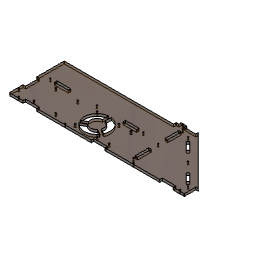
Side Plate Left (Autodesk Fusion 360 design; units mm, degrees)
Autodesk Fusion 360 part; units mm, degrees
note: some values were not read from the file. Set by a fixed rule: which sketch regions a step uses.
sketch "Sketch1" plane through (0, 0, 0) normal (0, 0, 1) x (1, 0, 0)
  line L0 (0, 0) -> (320, 0)
  line L1 (320, 0) -> (320, 10)
  line L2 (320, 10) -> (225, 105)
  line L3 (225, 105) -> (200, 105)
  line L4 (200, 105) -> (200, 100.25)
  line L5 (200, 100.25) -> (0, 100.25)
  line L6 (0, 100.25) -> (0, 0)
  line L7 (-10, 62.25) -> (295, 62.25) construction
  line L8 (-10, 57.75) -> (295, 57.75) construction
  line L9 (-10, 4.5) -> (325, 4.5) construction
  line L10 (9.1552, 60) -> (314.1552, 60) construction
  line L11 (325.1257, 2.25) -> (-10, 2.25) construction
  line L12 (25, 105) -> (25, -5) construction
  line L13 (50, 105) -> (50, -5) construction
  line L14 (175, 105) -> (175, -5) construction
  line L15 (150, 105) -> (150, -5) construction
  line L16 (4.5, 110) -> (4.5, -5) construction
  line L17 (150, 62.25) -> (175, 62.25)
  line L18 (175, 62.25) -> (175, 57.75)
  line L19 (175, 57.75) -> (150, 57.75)
  line L20 (150, 57.75) -> (150, 62.25)
  line L21 (25, 62.25) -> (50, 62.25)
  line L22 (50, 62.25) -> (50, 57.75)
  line L23 (50, 57.75) -> (25, 57.75)
  line L24 (25, 57.75) -> (25, 62.25)
  line L25 (25, 4.5) -> (50, 4.5)
  line L26 (50, 4.5) -> (50, 0)
  line L27 (50, 0) -> (25, 0)
  line L28 (25, 0) -> (25, 4.5)
  line L29 (150, 4.5) -> (175, 4.5)
  line L30 (175, 4.5) -> (175, 0)
  line L31 (175, 0) -> (150, 0)
  line L32 (150, 0) -> (150, 4.5)
  line L33 (300, -5) -> (300, 105) construction
  line L34 (275, 105) -> (275, -5) construction
  line L35 (275, 4.5) -> (300, 4.5)
  line L36 (300, 4.5) -> (300, 0)
  line L37 (300, 0) -> (275, 0)
  line L38 (275, 0) -> (275, 4.5)
  line L39 (0, 25) -> (4.5, 25)
  line L40 (4.5, 25) -> (4.5, 50)
  line L41 (4.5, 50) -> (0, 50)
  line L42 (0, 50) -> (0, 25)
  line L43 (215, 110) -> (215, -5) construction
  line L44 (219.5, 110) -> (219.5, -5) construction
  line L45 (250, 95) -> (182.1863, 95) construction
  line L46 (250, 70) -> (182.1863, 70) construction
  line L47 (250, 15) -> (182.1863, 15) construction
  line L48 (250, 40) -> (182.1863, 40) construction
  line L49 (219.5, 15) -> (215, 15)
  line L50 (215, 15) -> (215, 40)
  line L51 (215, 40) -> (219.5, 40)
  line L52 (219.5, 40) -> (219.5, 15)
  line L53 (219.5, 70) -> (215, 70)
  line L54 (215, 70) -> (215, 95)
  line L55 (215, 95) -> (219.5, 95)
  line L56 (219.5, 95) -> (219.5, 70)
  line L57 (217.25, 110) -> (217.25, -5) construction
  circle A0 centre (217.25, 100) radius 1.15
  circle A1 centre (217.25, 55) radius 1.15
  circle A2 centre (217.25, 10) radius 1.15
  circle A3 centre (185, 60) radius 1.15
  circle A4 centre (100, 60) radius 1.15
  circle A5 centre (15, 60) radius 1.15
  circle A6 centre (15, 2.25) radius 1.15
  circle A7 centre (100, 2.25) radius 1.15
  circle A8 centre (225, 2.25) radius 1.15
  circle A9 centre (310, 2.25) radius 1.15
  line L58 (329.3164, -5.6804) -> (209.3319, 114.3041) construction
  line L59 (242.2183, 87.7817) -> (239.0363, 84.5998)
  line L60 (256.3604, 73.6396) -> (253.1784, 70.4576)
  line L61 (291.7157, 38.2843) -> (288.5337, 35.1023)
  line L62 (305.8579, 24.1421) -> (302.6759, 20.9602)
  line L63 (239.0363, 84.5998) -> (253.1784, 70.4576)
  line L64 (288.5337, 35.1023) -> (302.6759, 20.9602)
  line L65 (330.1331, -3.3151) -> (213.3936, 113.4244) construction
  circle A10 centre (311.3379, 15.4801) radius 1.15
  circle A11 centre (272.4471, 54.371) radius 1.15
  circle A12 centre (233.5562, 93.2618) radius 1.15
  line L66 (2.25, -5) -> (2.25, 105) construction
  circle A13 centre (2.25, 15) radius 1.15
  line L67 (204.9, 105) -> (214.9, 105)
  line L68 (214.9, 105) -> (214.9, 109.5)
  line L69 (214.9, 109.5) -> (204.9, 109.5)
  line L70 (204.9, 109.5) -> (204.9, 105)
  line L71 (204.9, 107.25) -> (215.1, 107.25) construction
  circle A14 centre (210, 107.25) radius 1.15
  line L72 (236, 105) -> (225, 105)
  line L73 (236, 105) -> (236, 109.5)
  line L74 (320, 0) -> (331, 0)
  line L75 (331, 0) -> (331, 10)
  line L76 (331, 10) -> (331, 14.5)
  line L77 (331, 14.5) -> (236, 109.5)
  line L78 (320, 10) -> (320, 25.5)
  line L79 (340, 30) -> (285, 30)
  line L80 (75, 10) -> (35, 10) construction
  line L81 (35, 10) -> (35, 50) construction
  line L82 (35, 50) -> (75, 50) construction
  line L83 (75, 50) -> (75, 10) construction
  line L84 (75, 10) -> (35, 50) construction
  line L85 (35, 10) -> (75, 50) construction
  circle A15 centre (75, 50) radius 1.45
  circle A16 centre (75, 10) radius 1.45
  circle A17 centre (35, 50) radius 1.45
  circle A18 centre (35, 10) radius 1.45
  line L86 (320, 21) -> (324.5, 21)
  line L87 (155, 5.5) -> (105, 5.5) construction
  line L88 (105, 5.5) -> (105, 55.5) construction
  line L89 (105, 55.5) -> (155, 55.5) construction
  line L90 (155, 55.5) -> (155, 5.5) construction
  line L91 (155, 5.5) -> (105, 55.5) construction
  line L92 (105, 5.5) -> (155, 55.5) construction
  line L93 (150, 10.5) -> (110, 10.5) construction
  line L94 (110, 10.5) -> (110, 50.5) construction
  line L95 (110, 50.5) -> (150, 50.5) construction
  line L96 (150, 50.5) -> (150, 10.5) construction
  line L97 (150, 10.5) -> (110, 50.5) construction
  line L98 (110, 10.5) -> (150, 50.5) construction
  circle A19 centre (150, 50.5) radius 1.6
  circle A20 centre (110, 50.5) radius 1.6
  circle A21 centre (150, 10.5) radius 1.6
  circle A22 centre (110, 10.5) radius 1.6
  circle A23 centre (130, 30.5) radius 12.5
  circle A24 centre (130, 30.5) radius 23.5
  line L99 (132.5, 35.5) -> (127.5, 35.5)
  line L100 (127.5, 35.5) -> (127.5, 55.5)
  line L101 (127.5, 55.5) -> (132.5, 55.5)
  line L102 (132.5, 55.5) -> (132.5, 35.5)
  line L103 (132.5, 35.5) -> (127.5, 55.5) construction
  line L104 (127.5, 35.5) -> (132.5, 55.5) construction
  line L105 (107.0994, 20.1651) -> (124.4199, 30.1651)
  line L106 (109.5994, 15.8349) -> (107.0994, 20.1651)
  line L107 (126.9199, 25.8349) -> (109.5994, 15.8349)
  line L108 (124.4199, 30.1651) -> (126.9199, 25.8349)
  line L109 (124.4199, 30.1651) -> (109.5994, 15.8349) construction
  line L110 (126.9199, 25.8349) -> (107.0994, 20.1651) construction
  line L111 (150.4006, 15.8349) -> (133.0801, 25.8349)
  line L112 (152.9006, 20.1651) -> (150.4006, 15.8349)
  line L113 (135.5801, 30.1651) -> (152.9006, 20.1651)
  line L114 (133.0801, 25.8349) -> (135.5801, 30.1651)
  line L115 (133.0801, 25.8349) -> (152.9006, 20.1651) construction
  line L116 (135.5801, 30.1651) -> (150.4006, 15.8349) construction
  line L117 (183.5, 7) -> (160.5, 7) construction
  line L118 (160.5, 7) -> (160.5, 54) construction
  line L119 (160.5, 54) -> (183.5, 54) construction
  line L120 (183.5, 54) -> (183.5, 7) construction
  line L121 (183.5, 7) -> (160.5, 54) construction
  line L122 (160.5, 7) -> (183.5, 54) construction
  line L123 (172, 62) -> (172, 11) construction
  circle A25 centre (172, 50.5) radius 1.6
  circle A26 centre (172, 10.5) radius 1.6
  point P0 (55, 30)
  point P1 (130, 30.5)
  point P2 (130, 30.5)
  point P3 (130, 45.5)
  point P4 (172, 30.5)
  dimension "d2" = 38
  dimension "d3" = 4.5
  dimension "d4" = 4.5
  dimension "d5" = 2.25
  dimension "d6" = 2.25
  dimension "d7" = 4.5
  dimension "d8" = 25
  dimension "d11" = 200
  dimension "d12" = 15
  dimension "d13" = 4.5
  dimension "d15" = 2.25
  dimension "d16" = 2.3
  dimension "d17" = 2.3
  dimension "d18" = 2.3
  dimension "d19" = 15
  dimension "d20" = 5
  dimension "d21" = 5
  dimension "d22" = 2.3
  dimension "d23" = 10
  dimension "d24" = 2.3
  dimension "d25" = 2.3
  dimension "d26" = 10
  dimension "d27" = 50
  dimension "d28" = 2.3
  dimension "d29" = 2.3
  dimension "d30" = 2.3
  dimension "d31" = 50
  dimension "d32" = 50
  dimension "d33" = 10
  dimension "d34" = 2.3
  dimension "d35" = 10
  dimension "d36" = 4.5
  dimension "d37" = 20
  dimension "d38" = 20
  dimension "d41" = 10
  dimension "d42" = 20
  dimension "d43" = 120
  dimension "d44" = 50
  dimension "d45" = 2.25
  dimension "d46" = 2.3
  dimension "d47" = 2.3
  dimension "d48" = 2.3
  dimension "d49" = 10
  dimension "d50" = 10
  dimension "d51" = 25
  dimension "d52" = 2.25
  dimension "d53" = 2.3
  dimension "d65" = 25
  dimension "d66" = 15
  dimension "d68" = 60
  dimension "d78" = 10
  dimension "d79" = 4.5
  dimension "d80" = 2.3
  dimension "d83" = 10
  dimension "d84" = 4.5
  dimension "d85" = 10
  dimension "d86" = 4.5
  dimension "d89" = 30
  dimension "d92" = 40
  dimension "d93" = 40
  dimension "d94" = 30
  dimension "d95" = 55
  dimension "d96" = 2.9
  dimension "d97" = 2.9
  dimension "d98" = 2.9
  dimension "d99" = 2.9
  dimension "d100" = 11
  dimension "d101" = 135
  dimension "d104" = 4.5
  dimension "d105" = 50
  dimension "d106" = 50
  dimension "d107" = 26
  dimension "d108" = 30
  dimension "d109" = 40
  dimension "d110" = 40
  dimension "d111" = 3.2
  dimension "d112" = 3.2
  dimension "d113" = 3.2
  dimension "d114" = 3.2
  dimension "d115" = 25
  dimension "d116" = 47
  dimension "d117" = 5
  dimension "d118" = 20
  dimension "d120" = 360
  dimension "d121" = 23
  dimension "d122" = 47
  dimension "d123" = 42
  dimension "d124" = 3.2
  dimension "d125" = 3.2
  dimension "d126" = 20
  dimension "d127" = 20
  constraint coincident L0.start L6.end
  constraint horizontal L0
  constraint perpendicular L0 L1
  constraint parallel L0 L3
  constraint perpendicular L3 L4
  constraint perpendicular L4 L5
  constraint perpendicular L0 L6
  constraint horizontal L7
  constraint horizontal L8
  constraint parallel L0 L9
  constraint parallel L8 L10
  constraint parallel L9 L11
  constraint perpendicular L5 L12
  constraint perpendicular L5 L13
  constraint perpendicular L11 L14
  constraint perpendicular L5 L15
  constraint perpendicular L9 L16
  constraint horizontal L17
  constraint vertical L18
  constraint horizontal L19
  constraint vertical L20
  constraint coincident L14 L18.end
  constraint coincident L8 L18.end
  constraint coincident L15 L17.start
  constraint coincident L7 L17.start
  constraint horizontal L21
  constraint vertical L22
  constraint horizontal L23
  constraint vertical L24
  constraint coincident L8 L22.end
  constraint coincident L13 L22.end
  constraint coincident L12 L21.start
  constraint coincident L7 L21.start
  constraint horizontal L25
  constraint vertical L26
  constraint horizontal L27
  constraint vertical L28
  constraint coincident L13 L26.end
  constraint coincident L0 L26.end
  constraint coincident L12 L25.start
  constraint coincident L9 L25.start
  constraint horizontal L29
  constraint vertical L30
  constraint horizontal L31
  constraint vertical L32
  constraint coincident L0 L30.end
  constraint coincident L14 L30.end
  constraint coincident L15 L29.start
  constraint coincident L9 L29.start
  constraint perpendicular L11 L33
  constraint perpendicular L0 L34
  constraint horizontal L35
  constraint vertical L36
  constraint horizontal L37
  constraint vertical L38
  constraint coincident L33 L36.end
  constraint coincident L0 L36.end
  constraint coincident L34 L35.start
  constraint coincident L9 L35.start
  constraint horizontal L39
  constraint vertical L40
  constraint horizontal L41
  constraint vertical L42
  constraint coincident L6 L39.start
  constraint perpendicular L0 L43
  constraint perpendicular L0 L44
  constraint perpendicular L43 L45
  constraint perpendicular L43 L46
  constraint perpendicular L43 L47
  constraint perpendicular L44 L48
  constraint horizontal L49
  constraint vertical L50
  constraint horizontal L51
  constraint vertical L52
  constraint coincident L43 L50.end
  constraint coincident L48 L50.end
  constraint coincident L44 L49.start
  constraint coincident L47 L49.start
  constraint horizontal L53
  constraint vertical L54
  constraint horizontal L55
  constraint vertical L56
  constraint coincident L45 L54.end
  constraint coincident L43 L54.end
  constraint coincident L46 L53.start
  constraint coincident L44 L53.start
  constraint parallel L43 L57
  constraint coincident L57 A0.centre
  constraint coincident L57 A1.centre
  constraint coincident L57 A2.centre
  constraint coincident L10 A3.centre
  constraint coincident L10 A4.centre
  constraint coincident L10 A5.centre
  constraint coincident L11 A6.centre
  constraint coincident L11 A7.centre
  constraint coincident L11 A8.centre
  constraint coincident L11 A9.centre
  constraint parallel L2 L58
  constraint coincident L2 L59.start
  constraint coincident L58 L59.end
  constraint perpendicular L58 L59
  constraint coincident L2 L60.start
  constraint coincident L58 L60.end
  constraint perpendicular L58 L60
  constraint coincident L2 L61.start
  constraint coincident L58 L61.end
  constraint perpendicular L58 L61
  constraint coincident L2 L62.start
  constraint coincident L58 L62.end
  constraint perpendicular L58 L62
  constraint parallel L58 L65
  constraint coincident L65 A10.centre
  constraint coincident L65 A11.centre
  constraint coincident L65 A12.centre
  constraint perpendicular L0 L66
  constraint coincident L66 A13.centre
  constraint horizontal L67
  constraint vertical L68
  constraint horizontal L69
  constraint vertical L70
  constraint coincident L3 L67.start
  constraint midpoint L70 L71.start
  constraint perpendicular L70 L71
  constraint midpoint L71 A14.centre
  constraint perpendicular L72 L73
  constraint perpendicular L1 L74
  constraint perpendicular L74 L75
  constraint parallel L75 L76
  constraint coincident L77 L78.end
  constraint parallel L1 L78
  constraint perpendicular L33 L79
  constraint horizontal L80
  constraint perpendicular L80 L81
  constraint parallel L80 L82
  constraint parallel L81 L83
  constraint coincident L84 P0
  constraint coincident L85 P0
  constraint coincident L82.end L83.start
  constraint coincident L80.start L83.end
  constraint coincident L81.end L82.start
  constraint coincident L80.end L81.start
  constraint collinear L3 L72
  constraint coincident L78 L86.start
  constraint perpendicular L78 L86
  constraint horizontal L87
  constraint perpendicular L87 L88
  constraint parallel L87 L89
  constraint parallel L88 L90
  constraint coincident L91 P2
  constraint coincident L92 P2
  constraint horizontal L93
  constraint perpendicular L93 L94
  constraint parallel L93 L95
  constraint parallel L94 L96
  constraint coincident L97 P2
  constraint coincident L98 P2
  constraint coincident P2 P1
  constraint coincident L95.end L96.start
  constraint coincident L94.end L95.start
  constraint coincident L93.start L96.end
  constraint coincident L93.end L94.start
  constraint concentric A23 A24
  constraint horizontal L99
  constraint perpendicular L99 L100
  constraint parallel L99 L101
  constraint parallel L100 L102
  constraint coincident L103 P3
  constraint coincident L104 P3
  constraint collinear L89 L101
  constraint horizontal L117
  constraint perpendicular L117 L118
  constraint parallel L117 L119
  constraint parallel L118 L120
  constraint coincident L121 P4
  constraint coincident L122 P4
  constraint perpendicular L117 L123
  constraint coincident P4 L123
  constraint coincident L123 A25.centre
  constraint coincident L123 A26.centre
  measures "d2" distance of L5 L7
  measures "d3" distance of L7 L8
  measures "d4" distance of L0 L9
  measures "d5" distance of L7 L10
  measures "d6" distance of L9 L11
  measures "d7" distance of L6 L16
  measures "d8" distance of L39.start L41.end
  measures "d11" distance of L4.end L5.end
  measures "d12" distance of L4 L43
  measures "d13" distance of L43 L44
  measures "d15" distance of L43 L57
  measures "d16" diameter of A0
  measures "d17" diameter of A1
  measures "d18" diameter of A2
  measures "d19" distance of L48 A1.centre
  measures "d20" distance of L45 A0.centre
  measures "d21" distance of L47 A2.centre
  measures "d22" diameter of A3
  measures "d23" distance of L14 A3.centre
  measures "d24" diameter of A4
  measures "d25" diameter of A5 L31.end
  measures "d26" distance of L12 A5.centre
  measures "d27" distance of L13 A4.centre
  measures "d28" diameter of A6
  measures "d29" diameter of A7
  measures "d30" diameter of A8
  measures "d31" distance of L14 A8.centre
  measures "d32" distance of L13 A7.centre
  measures "d33" distance of L12 A6.centre
  measures "d34" diameter of A9
  measures "d35" distance of L33 A9.centre
  measures "d36" distance of L2 L58
  measures "d37" distance of L59 L60
  measures "d38" distance of L61 L62
  measures "d41" distance of L0.end L1.end
  measures "d42" distance of L1.end L62.start
  measures "d43" distance of L1 L4
  measures "d44" distance of L60.start L61.start
  measures "d45" distance of L2 L65
  measures "d46" diameter of A10
  measures "d47" diameter of A11
  measures "d48" diameter of A12
  measures "d49" distance of L62 A10.centre
  measures "d50" distance of L59 A12.centre
  measures "d51" distance of L61 A11.centre
  measures "d52" distance of L6 L66
  measures "d53" diameter of A13
  measures "d65" distance of L0 L39
  measures "d66" distance of L0 A13.centre
  measures "d68" distance of L0 L10
  measures "d78" distance of L67.start L67.end
  measures "d79" distance of L67.start L69.end
  measures "d80" diameter of A14
  measures "d83" distance of L4 A14.centre
  measures "d84" distance of L72.start L73.end
  measures "d85" distance of L74.end L75.end
  measures "d86" distance of L75.end L76.end
  measures "d89" distance of L74 L79
  measures "d92" distance of L81.end L82.end
  measures "d93" distance of L80.end L81.end
  measures "d94" distance of L0 P0
  measures "d95" distance of L6 P0
  measures "d96" diameter of A15
  measures "d97" diameter of A16
  measures "d98" diameter of A17
  measures "d99" diameter of A18
  measures "d100" distance of L2.end L72.start
  measures "d101" angle of L76 L77
  measures "d104" distance of L78.end L86.start
  measures "d105" distance of L88.end L89.end
  measures "d106" distance of L87.end L88.end
  measures "d107" distance of L9 P2
  measures "d108" distance of L83 L88
  measures "d109" distance of L94.end L95.end
  measures "d110" distance of L93.end L94.end
  measures "d111" diameter of A19
  measures "d112" diameter of A20
  measures "d113" diameter of A21
  measures "d114" diameter of A22
  measures "d115" diameter of A23
  measures "d116" diameter of A24
  measures "d117" distance of L100.end L101.end
  measures "d118" distance of L99.end L100.end
  measures "d121" distance of L118.end L119.end
  measures "d122" distance of L117.end L118.end
  measures "d123" distance of P2 P4
  measures "d124" diameter of A25
  measures "d125" diameter of A26
  measures "d126" distance of P4 A25.centre
  measures "d127" distance of P4 A26.centre
extrude "Extrude1" add sketch "Sketch1" along normal blind 4.5 contours L0 L1 L2 L3 L4 L5 L6 L25 L26 L28 L29 L30 L32 L35 L36 L38 L39 L40 L41 L59 L60 L61 L62 L63 L64 L67 | L3 L67 L68 L69 L70 | L2 L77 L78 L79 | L2 L72 L73 L77 L79 | L77 L78 L86 | A23 L99 L100 L102 L105 L107 L108 L111 L113 L114 | A23 L99 L100 L102 | A23 A24 L100 L102 | A23 A24 L111 L113 | A23 L111 L113 L114 | A24 L100 L101 L102 | A24 L111 L112 L113 | A23 L105 L107 L108 | A23 A24 L105 L107 | A24 L105 L106 L107
fillet "Fillet1" radius 0.5 6 edges at (320, 0, 2.25) (320, 10, 2.25) (225, 105, 2.25) (200, 105, 2.25) (0, 100.25, 2.25) (0, 0, 2.25)
sketch "Sketch2" plane through (0, 0, 4.5) normal (0, 0, 1) x (-1, 0, 0)
  arc A0 (0, -0.5) -> (-0.5, 0) centre (-0.5, -0.5) ccw
  line L0 (-0.5, 0) -> (-25, 0)
  line L1 (-25, 0) -> (-25, -4.5)
  line L2 (-25, -4.5) -> (-50, -4.5)
  line L3 (-50, -4.5) -> (-50, 0)
  line L4 (-50, 0) -> (-150, 0)
  line L5 (-150, 0) -> (-150, -4.5)
  line L6 (-150, -4.5) -> (-175, -4.5)
  line L7 (-175, -4.5) -> (-175, 0)
  line L8 (-175, 0) -> (-275, 0)
  line L9 (-275, 0) -> (-275, -4.5)
  line L10 (-275, -4.5) -> (-300, -4.5)
  line L11 (-300, -4.5) -> (-300, 0)
  line L12 (-300, 0) -> (-319.5, 0)
  line L13 (-305.8579, -24.1421) -> (-302.6759, -20.9602)
  line L14 (-302.6759, -20.9602) -> (-288.5338, -35.1023)
  line L15 (-288.5338, -35.1023) -> (-291.7157, -38.2843)
  line L16 (-291.7157, -38.2843) -> (-305.8579, -24.1421)
  line L17 (-256.3604, -73.6396) -> (-253.1784, -70.4576)
  line L18 (-253.1784, -70.4576) -> (-239.0363, -84.5998)
  line L19 (-239.0363, -84.5998) -> (-242.2183, -87.7818)
  line L20 (-242.2183, -87.7818) -> (-256.3604, -73.6396)
  arc A1 (-200.5, -105) -> (-200, -104.5) centre (-200.5, -104.5) ccw
  line L21 (-200, -104.5) -> (-200, -100.25)
  line L22 (-200, -100.25) -> (-0.5, -100.25)
  arc A2 (-0.5, -100.25) -> (0, -99.75) centre (-0.5, -99.75) ccw
  line L23 (0, -99.75) -> (0, -50)
  line L24 (0, -50) -> (-4.5, -50)
  line L25 (-4.5, -50) -> (-4.5, -25)
  line L26 (-4.5, -25) -> (0, -25)
  line L27 (0, -25) -> (0, -0.5)
  circle A3 centre (-100, -2.25) radius 1.15
  line L28 (-50, -57.75) -> (-25, -57.75)
  line L29 (-25, -57.75) -> (-25, -62.25)
  line L30 (-25, -62.25) -> (-50, -62.25)
  line L31 (-50, -62.25) -> (-50, -57.75)
  circle A4 centre (-311.3379, -15.4801) radius 1.15
  circle A5 centre (-310, -2.25) radius 1.15
  circle A6 centre (-15, -60) radius 1.15
  circle A7 centre (-15, -2.25) radius 1.15
  line L32 (-215, -95) -> (-219.5, -95)
  line L33 (-219.5, -95) -> (-219.5, -70)
  line L34 (-219.5, -70) -> (-215, -70)
  line L35 (-215, -70) -> (-215, -95)
  circle A8 centre (-217.25, -55) radius 1.15
  circle A9 centre (-272.4471, -54.371) radius 1.15
  circle A10 centre (-233.5562, -93.2618) radius 1.15
  circle A11 centre (-217.25, -100) radius 1.15
  circle A12 centre (-100, -60) radius 1.15
  circle A13 centre (-217.25, -10) radius 1.15
  circle A14 centre (-185, -60) radius 1.15
  line L36 (-215, -40) -> (-219.5, -40)
  line L37 (-219.5, -40) -> (-219.5, -15)
  line L38 (-219.5, -15) -> (-215, -15)
  line L39 (-215, -15) -> (-215, -40)
  circle A15 centre (-225, -2.25) radius 1.15
  circle A16 centre (-2.25, -15) radius 1.15
  line L40 (-175, -57.75) -> (-150, -57.75)
  line L41 (-150, -57.75) -> (-150, -62.25)
  line L42 (-150, -62.25) -> (-175, -62.25)
  line L43 (-175, -62.25) -> (-175, -57.75)
  line L44 (-35, -30) -> (-187.4214, -30) construction
  line L45 (-187.4214, -30) -> (-187.4214, -58.9235) construction
  line L46 (-187.4214, -58.9235) -> (-35, -58.9235) construction
  line L47 (-35, -58.9235) -> (-35, -30) construction
  line L48 (-214.9, -105) -> (-214.9, -109.5)
  line L49 (-214.9, -109.5) -> (-204.9, -109.5)
  line L50 (-204.9, -109.5) -> (-204.9, -105)
  line L51 (-204.9, -105) -> (-200.5, -105)
  circle A17 centre (-210, -107.25) radius 1.15
  line L52 (-324.5, -21) -> (-236, -109.5)
  line L53 (-236, -109.5) -> (-236, -105)
  line L54 (-236, -105) -> (-214.9, -105)
  arc A18 (-319.5, 0) -> (-320, -0.5) centre (-319.5, -0.5) ccw
  line L55 (-320, -0.5) -> (-320, -21)
  circle A19 centre (-35, -50) radius 1.45
  circle A20 centre (-35, -10) radius 1.45
  circle A21 centre (-75, -10) radius 1.45
  circle A22 centre (-75, -50) radius 1.45
  line L56 (-320, -21) -> (-324.5, -21)
  circle A23 centre (-110, -10.5) radius 1.6
  circle A24 centre (-172, -10.5) radius 1.6
  circle A25 centre (-172, -50.5) radius 1.6
  circle A26 centre (-150, -10.5) radius 1.6
  circle A27 centre (-110, -50.5) radius 1.6
  circle A28 centre (-150, -50.5) radius 1.6
  line L57 (-127.5, -53.8666) -> (-127.5, -42.7474)
  arc A29 (-127.5, -42.7474) -> (-118.1434, -26.5413) centre (-130, -30.5) ccw
  line L58 (-118.1434, -26.5413) -> (-108.5139, -20.9817)
  arc A30 (-127.5, -53.8666) -> (-108.5139, -20.9817) centre (-130, -30.5) ccw
  line L59 (-111.0139, -16.6516) -> (-120.6434, -22.2112)
  arc A31 (-120.6434, -22.2112) -> (-139.3566, -22.2112) centre (-130, -30.5) ccw
  line L60 (-139.3566, -22.2112) -> (-148.9861, -16.6516)
  arc A32 (-111.0139, -16.6516) -> (-148.9861, -16.6516) centre (-130, -30.5) ccw
  arc A33 (-151.4861, -20.9817) -> (-132.5, -53.8666) centre (-130, -30.5) ccw
  line L61 (-151.4861, -20.9817) -> (-141.8566, -26.5413)
  arc A34 (-141.8566, -26.5413) -> (-132.5, -42.7474) centre (-130, -30.5) ccw
  line L62 (-132.5, -42.7474) -> (-132.5, -53.8666)
  dimension "d69" = 20
move_face "OffsetFaces1" offset -0.1 1 faces at (204.9, 108, 1.5)
fillet "Fillet2" radius 0.2 1 edges at (236, 109.5, 2.25)
fillet "Fillet3" [no effect]
equation "ScrewHole = 2.3 mm"
equation "d16 = ScrewHole"
equation "d17 = ScrewHole"
equation "d18 = ScrewHole"
equation "d22 = ScrewHole"
equation "d24 = ScrewHole"
equation "d25 = ScrewHole"
equation "d28 = ScrewHole"
equation "d29 = ScrewHole"
equation "d30 = ScrewHole"
equation "d34 = ScrewHole"
equation "d46 = ScrewHole"
equation "d47 = ScrewHole"
equation "d48 = ScrewHole"
equation "d53 = ScrewHole"
equation "TabRelief = -0.1 mm"
equation "d82 = TabRelief"
